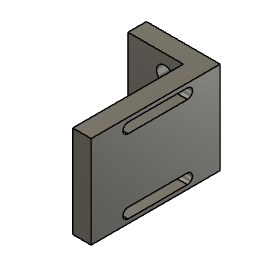
LaserSaftyInterlock v2 (Autodesk Fusion 360 design; units mm, degrees)
Autodesk Fusion 360 part; units mm, degrees
sketch "Sketch1" plane through (0, 0, 0) normal (0, 0, 1) x (1, 0, 0)
  line L0 (5, 5) -> (-5, 5)
  line L1 (-5, 5) -> (-5, -5)
  line L2 (-5, -5) -> (5, -5)
  line L3 (5, -5) -> (5, 5)
  line L4 (5, 5) -> (-5, -5) construction
  line L5 (-5, 5) -> (5, -5) construction
  line L6 (-5, 5) -> (5, 5)
  line L7 (5, 5) -> (5, 25)
  line L8 (5, 25) -> (-5, 25)
  line L9 (-5, 25) -> (-5, 5)
  circle A0 centre (0, 15) radius 4.5
  line L10 (-5, -15) -> (5, -15) construction
  line L11 (0, 25) -> (0, 5) construction
  line L12 (-5, 15) -> (5, 15) construction
  line L13 (20, 0) -> (2.5, 0) construction
  line L14 (5, -25) -> (-5, -25)
  line L15 (5, -5) -> (5, -25)
  line L16 (-5, -25) -> (-5, -5)
  circle A1 centre (0, -15) radius 4.5
  dimension "d1" = 10
  dimension "d2" = 10
  dimension "d3" = 20
  dimension "d4" = 9
  dimension "d5" = 10
  dimension "d6" = 10
  constraint horizontal L0
  constraint perpendicular L0 L1
  constraint parallel L0 L2
  constraint parallel L1 L3
  constraint coincident L4 origin
  constraint coincident L5 origin
  constraint horizontal L6
  constraint vertical L7
  constraint horizontal L8
  constraint vertical L9
  constraint coincident L9 L10.start
  constraint coincident L7 L10.end
  constraint perpendicular L7 L10
  constraint midpoint L8 L11.start
  constraint midpoint L6 L11.end
  constraint symmetric L0 L8 L10
  constraint coincident L9 L12.start
  constraint coincident L7 L12.end
  constraint perpendicular L7 L12
  constraint coincident A0.centre L12
  constraint coincident A0.centre L11
  constraint symmetric L0.end L13 L1.end
  constraint symmetric L0.start L13 L2.end
  constraint symmetric L7.end L13 L14.start
  constraint symmetric L8.end L13 L14.end
  constraint symmetric A0 L13 A1
  measures "d1" distance of L1.end L2.end
  measures "d2" distance of L0.end L1.end
  measures "d3" distance of L0.end L8.end
  measures "d4" diameter of A0
  measures "d5" distance of L7 L9
  measures "d6" distance of L8 L12
extrude "Extrude1" add sketch "Sketch1" against normal blind 10 contours L0 L1 L2 L3 L6
extrude "Extrude2" add sketch "Sketch1" 1 faces at (-1.6667, -1.6667, 0) along normal blind 10 contours L0 L6 L7 L8 L9 | L2 L14 L15 L16
sketch "Sketch2" plane through (5, 0, 0) normal (1, 0, 0) x (0, 0, -1)
  line L0 (0, -5) -> (10, -5)
  line L1 (10, -5) -> (10, 5)
  line L2 (10, 5) -> (0, 5)
  line L3 (0, 5) -> (0, 25)
  line L4 (0, 25) -> (-10, 25)
  line L5 (-10, 25) -> (-10, -25)
  line L6 (-10, -25) -> (0, -25)
  line L7 (0, -25) -> (0, -5)
  line L8 (-10, 25) -> (0, 25)
  line L9 (0, 25) -> (0, -25)
  line L10 (0, -25) -> (-10, -25)
  line L11 (-10, -25) -> (-10, 25)
  constraint horizontal L8
  constraint vertical L9
  constraint horizontal L10
  constraint vertical L11
  constraint coincident L6.end L7.start
  constraint coincident L4.end L5.start
extrude "Extrude3" add sketch "Sketch2" along normal blind 15 contours L3 L4 L5 L6 L7 L8 L9 L10 L11
sketch "Sketch3" plane through (0, 0, 10) normal (0, 0, 1) x (1, 0, 0)
  circle A0 centre (0, -15) radius 4.5
  circle A1 centre (0, 15) radius 4.5
  line L0 (-5, 25) -> (-5, -25)
  line L1 (-5, -25) -> (20, -25)
  line L2 (20, -25) -> (20, 25)
  line L3 (20, 25) -> (-5, 25)
  line L4 (20, 25) -> (10, 25)
  line L5 (10, 25) -> (10, -25)
  line L6 (10, -25) -> (20, -25)
  line L7 (20, -25) -> (20, 25)
  constraint horizontal L4
  constraint vertical L5
  constraint horizontal L6
  constraint vertical L7
  constraint coincident L1 L5.end
  constraint coincident L2.end L3.start
extrude "Extrude4" add sketch "Sketch3" along normal blind 60 contours L1 L2 L3 L4 L5 L6 L7
sketch "Sketch4" plane through (20, 0, 0) normal (1, 0, 0) x (0, 0, -1)
  line L0 (-70, -25) -> (0, -25)
  line L1 (0, -25) -> (0, 25)
  line L2 (0, 25) -> (-70, 25)
  line L3 (-70, 25) -> (-70, -25)
  line L4 (-70, 0) -> (0, 0) construction
  circle A0 centre (-50, 20) radius 2.75
  circle A1 centre (-17.75, 20) radius 2.75
  line L5 (-50, 22.75) -> (-17.75, 22.75)
  line L6 (-17.75, 17.25) -> (-50, 17.25)
  line L7 (0, 5) -> (0, 25)
  circle A2 centre (-50, -20) radius 2.75
  line L8 (-50, -22.75) -> (-17.75, -22.75)
  line L9 (-17.75, -17.25) -> (-50, -17.25)
  circle A3 centre (-17.75, -20) radius 2.75
  dimension "d15" = 5.5
  dimension "d16" = 5.5
  dimension "d17" = 20
  dimension "d18" = 20
  dimension "d19" = 17.75
  dimension "d20" = 20
  constraint midpoint L3 L4.start
  constraint coincident L4.end origin
  constraint coincident A0 L5.start
  constraint coincident A1 L5.end
  constraint tangent A1 L5
  constraint coincident A1 L6.start
  constraint coincident A0 L6.end
  constraint tangent A0 L6
  constraint horizontal L6
  constraint tangent A1 L6
  constraint tangent A0 L5
  constraint parallel L5 L6
  constraint symmetric L4 A0 A2
  constraint symmetric L4 A1 A3
  constraint symmetric L4 L5.start L8.start
  constraint symmetric L4 L5.end L8.end
  constraint symmetric L4 L6.start L9.start
  constraint symmetric L4 L6.end L9.end
  measures "d15" diameter of A0
  measures "d16" diameter of A1
  measures "d17" distance of L4 A1.centre
  measures "d18" distance of L4 A0.centre
  measures "d19" distance of A1.centre L7
  measures "d20" distance of L3 A0.centre
extrude "Extrude5" cut sketch "Sketch4" against normal through all contours A0 | A0 A1 L5 L6 | A1 | A2 | A2 L8 L9 A3 | A3
sketch "Sketch5" plane through (-5, 0, 0) normal (-1, 0, 0) x (0, 0, 1)
  line L0 (0, 5) -> (-10, 5)
  line L1 (-10, 5) -> (-10, -5)
  line L2 (-10, -5) -> (0, -5)
  line L3 (0, -5) -> (0, -25)
  line L4 (0, -25) -> (10, -25)
  line L5 (10, -25) -> (10, 25)
  line L6 (10, 25) -> (0, 25)
  line L7 (0, 25) -> (0, 5)
  line L8 (0, 25) -> (10, 25)
  line L9 (10, 25) -> (10, -25)
  line L10 (10, -25) -> (0, -25)
  line L11 (0, -25) -> (0, 25)
  constraint horizontal L8
  constraint vertical L9
  constraint horizontal L10
  constraint vertical L11
  constraint coincident L4.end L5.start
  constraint coincident L6.end L7.start
extrude "Extrude6" add sketch "Sketch5" along normal blind 15 contours L3 L4 L5 L6 L7 L8 L9 L10 L11
equation "d19 = 10 mm + ( 5.5 / 2 ) * 1 mm + 5 mm"
